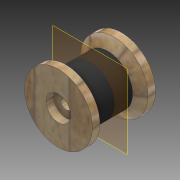
# Autodesk Inventor part: 1219_Middle Roller_V1
Saved by Autodesk Inventor 2020 (Build 240168000, 168)
## iProperties
Created: 2017-11-07
Part Number: 1219_Middle Roller_V1
Material: Wood (Maple)
Document SubType Name: Modeling
Designer: e22ma
Density: 0.67 g/cm^3
Appearance: Natural Maple - Glossy Dark Tint
Author: e22ma
Autodesk Inventor part; units mm, degrees
ref_plane "YZ Plane" through (0, 0, 0) normal (1, 0, 0) x (0, 1, 0)
ref_plane "XZ Plane" through (0, 0, 0) normal (0, 1, 0) x (-1, 0, 0)
ref_plane "XY Plane" through (0, 0, 0) normal (0, 0, 1) x (1, 0, 0)
sketch "Sketch1" plane through (0, 0, 0) normal (0, 0, 1) x (1, 0, 0)
  line L0 (0, 0) -> (0, 58)
  line L1 (0, 58) -> (20, 58)
  line L2 (20, 58) -> (20, 0)
  line L3 (20, 0) -> (0, 0)
  line L4 (40, 0) -> (40, 58)
  line L5 (40, 58) -> (55, 68)
  line L6 (55, 68) -> (55, 80.225)
  line L7 (55, 80.225) -> (20, 80.225)
  line L8 (20, 80.225) -> (20, -22.225)
  line L9 (20, -22.225) -> (55, -22.225)
  line L10 (55, -22.225) -> (55, -10)
  line L11 (55, -10) -> (40, 0)
  line L12 (20, 0) -> (8.5, 0)
  line L13 (8.5, 0) -> (8.5, 58)
  line L14 (8.5, 58) -> (20, 58)
  line L15 (20, 58) -> (20, 0)
  line L16 (8.5, -9.725) -> (20, -9.725)
  line L17 (20, -9.725) -> (20, 67.725)
  line L18 (20, 67.725) -> (8.5, 67.725)
  line L19 (8.5, 67.725) -> (8.5, -9.725)
  dimension "d0" = 58
  dimension "d1" = 20
  dimension "d9" = 12.225
  dimension "d10" = 10
  dimension "d14" = 8.5
  dimension "d15" = 102.45
  dimension "d16" = 77.45
  dimension "d17" = 12.5
  dimension "d18" = 35
  dimension "d19" = 40
  dimension "d20" = 35
  dimension "d21" = 12.225
  dimension "d22" = 10
  constraints: 40 end point, 7 perpendicular, 6 parallel, 3 horizontal, 3 point on line, 2 horizontal alignment, 2 vertical, 1 collinear
  measures "d0" distance of L0.start L0.end
  measures "d1" distance of L0.end L1.end
  measures "d9" distance of L9.end L10.end
  measures "d10" vertical distance of L10.end L4.start
  measures "d14" distance between parallel lines of L13 L0
  measures "d15" distance between parallel lines of L7 L9
  measures "d16" distance between parallel lines of L18 L16
  measures "d17" distance between parallel lines of L9 L16
  measures "d18" distance of L8.end L9.end
  measures "d19" distance between parallel lines of L0 L4
  measures "d20" distance of L6.end L7.end
  measures "d21" distance of L5.end L6.end
  measures "d22" vertical distance of L4.end L5.end
revolve "Revolution1" add sketch "Sketch1" angle 360 about axis through (0, 0, 0) along (0, 1, 0) contours L13 L1 L2 L3 | L3 L8 L16 L19 | L19 L18 L8 L1 | L2 L8 L7 L6 L5 L4 L11 L10 L9
ref_plane "Work Plane1" through (0, 29, 0) normal (0, -1, 0) x (1, 0, 0)
equation "\"d9\" = d5"
equation "\"d10\" = d7"
equation "\"d17\" = -0.5 * d16 + 0.5 * d15"
equation "\"d20\" = d18"
equation "\"d21\" = d9"
equation "\"d5\" = 12.225"
equation "\"d7\" = 10"
body "Solid1"
